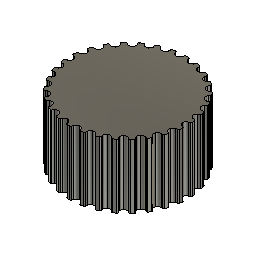
gear_30z (Autodesk Fusion 360 design; units mm, degrees)
Autodesk Fusion 360 part; units mm, degrees
sketch "Sketch1" plane through (0, 0, 0) normal (0, 0, 1) x (1, 0, 0) in component "gt2 pulley"
  circle A0 centre (0, 0) radius 9.5493 construction
  circle A1 centre (0, 0) radius 8.5453 construction
  line L0 (0, 0) -> (0, 9.5493) construction
  line L1 (0, 0) -> (0.9982, 9.497) construction
  line L2 (0, 0) -> (1.4102, 9.4446) construction
  circle A2 centre (0, 0) radius 9.2953 construction
  arc A3 (0.3736, 9.1492) -> (0.4257, 8.8722) centre (1.3727, 9.1934) ccw
  circle A4 centre (0, 0) radius 9.1453 construction
  arc A5 (0.2274, 9.2925) -> (0, 9.2953) centre (0, 0) ccw
  arc A6 (0.3736, 9.1492) -> (0.2274, 9.2925) centre (0.2238, 9.1426) ccw
  arc A7 (0.4257, 8.8722) -> (0.8932, 8.4985) centre (0.9512, 9.0504) ccw
  arc A8 (0, 9.2953) -> (-0.2274, 9.2925) centre (0, 0) ccw
  arc A9 (-0.2274, 9.2925) -> (-0.3736, 9.1492) centre (-0.2238, 9.1426) ccw
  arc A10 (-0.4257, 8.8722) -> (-0.3736, 9.1492) centre (-1.3727, 9.1934) ccw
  arc A11 (-0.893, 8.4985) -> (-0.4257, 8.8722) centre (-0.9512, 9.0504) ccw
  arc A12 (0.8932, 8.4985) -> (-0.8932, 8.4985) centre (0, 0) ccw
  point P0 (1.3727, 9.1934)
  point P1 (0, 9.2953)
  dimension "d18" = 19.0986
  dimension "d19" = 6
  dimension "d22" = 1.004
  dimension "d24" = 0.75
  dimension "d26" = 1
  dimension "d27" = 0.15
  dimension "d28" = 0.15
  dimension "d47" = 0.555
  dimension "d52" = 3.812
  constraint coincident A0.centre A1.centre
  constraint coincident A0 L0.end
  constraint vertical L0
  constraint coincident A0 L1.end
  constraint coincident A0 L2.end
  constraint concentric A1 A2
  constraint coincident A1 A7.end
  constraint coincident L1 A7.end
  constraint coincident A2 P0
  constraint coincident L2 P0
  constraint coincident P0 A3.centre
  constraint coincident A2 P1
  constraint coincident L0 P1
  constraint concentric A2 A4
  constraint coincident P1 A5.end
  constraint coincident A4 A6.centre
  constraint coincident A3.start A6.start
  constraint tangent A3 A6
  constraint tangent A3 A7
  constraint symmetric L0 A7.end A12.end
  constraint symmetric L0 A3.start A9.end
  constraint symmetric L0 A3.end A10.start
  constraint symmetric L0 A3 A10
  constraint symmetric L0 A5.start A8.end
  constraint symmetric L0 P1 A5.end
  constraint symmetric L0 A5 A8
  constraint symmetric L0 A6 A9
  constraint symmetric L0 A7 A11
  constraint coincident A1 A11.start
  constraint tangent A1 A7
  constraint coincident L1 A7.centre
  measures "d18" diameter of A0
  measures "d19" angle of L0 L1
  measures "d22" distance of A0 A1
  measures "d24" distance of A1 A2
  measures "d26" radius of A3
  measures "d27" distance of A2 A4
  measures "d28" radius of A6
  measures "d47" radius of A7
extrude "Extrude1" add sketch "Sketch1" along normal blind 10 makes body 1
pattern_circular "C-Pattern1" count 30 over 360 about axis through (0, 0, 1.75) along (0, 0, 1) of bodies 1 makes body 2 at (-2.4506, 8.1864, 6.6667) makes body 3 at (-2.829, 8.0634, 3.3333) makes body 4 at (-4.4437, 7.299, 3.3333) makes body 5 at (-6.7944, 5.1825, 6.6667) makes body 6 at (-7.7234, 3.6566, 6.6667) makes body 7 at (-8.2668, 2.1638, 6.6667) makes body 8 at (-8.5083, 0.7944, 6.6667) makes body 9 at (-8.543, -0.1988, 3.3333) makes body 10 at (-8.0958, -2.7349, 6.6667) makes body 11 at (-7.0284, -4.8604, 6.6667) makes body 12 at (-5.8643, -6.2155, 6.6667) makes body 13 at (-5.5686, -6.4817, 3.3333) makes body 14 at (-2.8292, -8.0633, 6.6667) makes body 15 at (-1.0909, -8.4754, 6.6667) makes body 16 at (0.695, -8.517, 6.6667) makes body 17 at (1.0907, -8.4754, 3.3333) makes body 18 at (2.829, -8.0634, 3.3333) makes body 19 at (4.4437, -7.299, 3.3333) makes body 20 at (6.7944, -5.1825, 6.6667) makes body 21 at (7.7234, -3.6566, 6.6667) makes body 22 at (8.2668, -2.1638, 6.6667) makes body 23 at (8.5083, -0.7944, 6.6667) makes body 24 at (8.3977, 1.5815, 6.6667) makes body 25 at (7.8854, 3.2929, 6.6667) makes body 26 at (7.0284, 4.8604, 6.6667) makes body 27 at (6.2835, 5.7913, 6.6667) makes body 28 at (4.4439, 7.2989, 6.6667) makes body 29 at (2.8292, 8.0633, 6.6667) makes body 30 at (2.4508, 8.1863, 3.3333)
sketch "Sketch2" plane through (0, 0, 10) normal (0, 0, 1) x (-1, 0, 0)
  arc A0 (-7.0492, -5.8443) -> (-7.0578, -6.0489) centre (-6.944, -5.9513) ccw
  arc A1 (-7.0578, -6.0489) -> (-6.7535, -6.3869) centre (0, 0) ccw
  arc A2 (-6.7535, -6.3869) -> (-6.5492, -6.3997) centre (-6.6445, -6.2839) ccw
  arc A3 (-6.3085, -6.253) -> (-6.5492, -6.3997) centre (-5.9135, -7.1717) ccw
  arc A4 (-5.7181, -6.3502) -> (-6.3085, -6.253) centre (-6.0893, -6.7628) ccw
  arc A5 (-6.9133, -5.0228) -> (-5.7181, -6.3502) centre (0, 0) ccw
  arc A6 (-6.8781, -5.6203) -> (-6.9133, -5.0228) centre (-7.3623, -5.349) ccw
  arc A7 (-7.0492, -5.8443) -> (-6.8781, -5.6203) centre (-7.7505, -5.1315) ccw
  circle A8 centre (0, 0) radius 8.5453
  constraint coincident A1.centre A5.centre
extrude "Extrude2" add sketch "Sketch2" against normal blind 10 contours A5 A8 bodies 1 2 3 4 5 6 7 8 9 10 11 12 13 14 15 16 17 18 19 20 21 22 23 24 25 26 27 28 29 30
extrude "Extrude4" [suppressed] in component "gt2 pulley"
pattern_circular "C-Pattern7" [suppressed] in component "gt2 pulley"
extrude "Extrude3" [suppressed] in component "gt2 pulley"
pattern_circular "C-Pattern6" [suppressed] in component "gt2 pulley"
extrude "Extrude2'" [suppressed] in component "gt2 pulley"
pattern_circular "C-Pattern5" [suppressed] in component "gt2 pulley"
extrude "Extrude1'" [suppressed] in component "gt2 pulley"
pattern_circular "C-Pattern4" [suppressed] in component "gt2 pulley"
pattern_circular "C-Pattern3" [suppressed] in component "gt2 pulley"
pattern_circular "C-Pattern2" [suppressed] in component "gt2 pulley"
pattern_circular "C-Pattern1'" [suppressed] in component "gt2 pulley"
copy_body "Body->Comp1" [suppressed] in component "Component"
copy_body "Body->Comp2" [suppressed] in component "Component'"
copy_body "Body->Comp3" [suppressed] in component "Component''"
copy_body "Body->Comp4" [suppressed] in component "Component'''"
copy_body "Body->Comp5" [suppressed] in component "Component''''"
copy_body "Body->Comp6" [suppressed] in component "Component'''''"
copy_body "Body->Comp7" [suppressed] in component "Component''''''"
copy_body "Body->Comp8" [suppressed] in component "Component'''''''"
copy_body "Body->Comp9" [suppressed] in component "Component''''''''"
copy_body "Body->Comp10" [suppressed] in component "Component'''''''''"
copy_body "Body->Comp11" [suppressed] in component "Component''''''''''"
copy_body "Body->Comp12" [suppressed] in component "Component'''''''''''"
copy_body "Body->Comp13" [suppressed] in component "Component''''''''''''"
copy_body "Body->Comp14" [suppressed] in component "Component'''''''''''''"
copy_body "Body->Comp15" [suppressed] in component "Component''''''''''''''"
copy_body "Body->Comp16" [suppressed] in component "Component'''''''''''''''"
copy_body "Body->Comp17" [suppressed] in component "Component''''''''''''''''"
copy_body "Body->Comp18" [suppressed] in component "Component'''''''''''''''''"
copy_body "Body->Comp19" [suppressed] in component "Component''''''''''''''''''"
copy_body "Body->Comp20" [suppressed] in component "Component'''''''''''''''''''"
component "gt2 pulley" placed x (1, 0, 0) y (0, 1, 0) z (0, 0, 1) at (0, 0, 0)
equation "NumTeeth = 30" comment "min 20"
equation "ToothPitch = 2 mm"
equation "PullyDia = NumTeeth * ToothPitch / PI"
equation "ToothAng = ( ( 360 / NumTeeth ) * 1 deg )"
equation "TransOffsetAngle = ToothAng * 0.2"
equation "Sholulder_Radius = 0.15 mm"
equation "Root_Radius = 0.555 mm"
equation "TransRadius = 1 mm"
equation "ToolHeight = 0.75 mm"
equation "PLD = 0.254 mm"
equation "d18 = PullyDia"
equation "d19 = ToothAng / 2"
equation "d22 = PLD + ToolHeight"
equation "d24 = ToolHeight"
equation "d26 = TransRadius"
equation "d27 = Sholulder_Radius"
equation "d31 = NumTeeth"
equation "d33 = NumTeeth"
equation "d35 = NumTeeth"
equation "d37 = NumTeeth"
equation "d41 = NumTeeth"
equation "d45 = NumTeeth"
equation "d47 = Root_Radius"
equation "d50 = NumTeeth"
